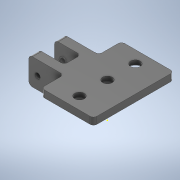
# Autodesk Inventor part: pulleysupport2
Saved by Autodesk Inventor 2020.2 (Build 242310000, 310)
## iProperties
Created: 2020-08-06
Part Number: pulleysupport2
Material: Generic
Document SubType Name: Modeling
Designer: JK
Density: 1 g/cm^3
Appearance: Smooth - Black
Author: JK
Autodesk Inventor part; units mm, degrees
sketch "Sketch1" plane through (0, 0, 0) normal (0, 1, 0) x (-1, 0, 0)
  line L0 (-15, 23) -> (15, 23)
  line L1 (15, 23) -> (15, -23)
  line L2 (15, -23) -> (-15, -23)
  line L3 (-15, -23) -> (-15, 23)
  line L4 (-15, 23) -> (15, -23) construction
  line L5 (15, 23) -> (-15, -23) construction
  circle A0 centre (0, 16) radius 1.75
  circle A1 centre (0, -16) radius 1.75
  point P0 (0, 0)
  dimension "d0" = 3.5
  dimension "d1" = 30
  dimension "d2" = 46
  dimension "d3" = 16
  dimension "d4" = 16
  constraints: 12 end point, 2 centre point, 2 midpoint, 2 parallel, 1 equal radius, 1 horizontal, 1 perpendicular
  measures "d0" diameter of A0
  measures "d1" distance of L0.start L0.end
  measures "d2" distance of L0.end L1.end
  measures "d3" distance of A0.centre point (0, 0)
  measures "d4" distance of A1.centre point (0, 0)
extrude "Extrusion1" add sketch "Sketch1" along normal blind 4
sketch "Sketch2" plane through (0, 4, 0) normal (0, 1, 0) x (1, 0, 0)
  line L0 (15, -23) -> (15, 23) projected
  line L1 (15, -10) -> (-35, -10)
  line L2 (-35, -10) -> (-35, 10)
  line L3 (-35, 10) -> (15, 10)
  line L4 (15, 10) -> (15, -10)
  line L5 (-15, -23) -> (15, -23) projected
  point P0 (0, 0)
  point P1 (15, 10)
  dimension "d9" = 20
  dimension "d11" = 10
  dimension "d28" = 50
  constraints: 8 end point, 2 parallel, 1 horizontal, 1 perpendicular, 1 point on line
  measures "d9" distance between parallel lines of L1 L3
  measures "d11" distance from line of L1 point (0, 0)
  measures "d28" distance between parallel lines of L0 L2
extrude "Extrusion2" add sketch "Sketch2" against normal blind 20
sketch "Sketch3" plane through (0, -16, 0) normal (0, -1, 0) x (1, 0, 0)
  point P0 (0, 0)
sketch "Sketch4" plane through (0, -16, 0) normal (0, -1, 0) x (1, 0, 0)
  line L0 (35.8206, -4.75) -> (-35.8206, -4.75)
  line L1 (-35.8206, -4.75) -> (-35.8206, 4.75)
  line L2 (-35.8206, 4.75) -> (35.8206, 4.75)
  line L3 (35.8206, 4.75) -> (35.8206, -4.75)
  line L4 (35.8206, -4.75) -> (-35.8206, 4.75) construction
  line L5 (-35.8206, -4.75) -> (35.8206, 4.75) construction
  point P0 (0, 0)
  dimension "d12" = 9.5
  constraints: 12 end point, 2 midpoint, 2 parallel, 1 horizontal, 1 perpendicular
  measures "d12" distance between parallel lines of L2 L0
extrude "Extrusion3" cut sketch "Sketch4" against normal up to surface (16 mm away)
sketch "Sketch5" plane through (-15, 4, -10) normal (0, 0, -1) x (-1, 0, 0)
  circle A0 centre (15, -8) radius 1.5
  line L0 (20, 0) -> (20, -20) projected
  line L1 (20, -20) -> (-30, -20) projected
  line L2 (20, 0) -> (0, 0) projected
  point P0 (-15, -4)
  dimension "d15" = 3
  dimension "d16" = 5
  dimension "d49" = 8
  constraints: 1 centre point
  measures "d15" diameter of A0
  measures "d16" distance from line of L0 A0.centre
  measures "d49" distance from line of A0.centre L2
extrude "Extrusion4" cut sketch "Sketch5" against normal through all
sketch "Sketch6" plane through (0, 0, 0) normal (0, -1, 0) x (1, 0, 0)
  circle A0 centre (0, -16) radius 1.75 projected
  circle A1 centre (0, -16) radius 4.75
  circle A2 centre (0, 16) radius 1.75 projected
  circle A3 centre (0, 16) radius 4.75
  point P0 (0, 0)
  dimension "d20" = 9.5
  dimension "d21" = 9.5
  constraints: 2 centre point, 2 coincident
  measures "d20" diameter of A1
  measures "d21" diameter of A3
extrude "Extrusion5" cut sketch "Sketch6" against normal blind 2
fillet "Fillet1" radius 2 6 edges at (-15, 2, -23) (15, 2, -23) (-15, 2, 23) (15, 2, 23) (-35, -16, -7.375) (-35, -16, 7.375)
chamfer "Chamfer1" distance 16 angle 45 2 edges at (15, -16, -7.375) (15, -16, 7.375)
fillet "Fillet2" radius 2 2 edges at (-1, -16, 7.375) (-1, -16, -7.375)
fillet "Fillet4" radius 2 2 edges at (0, 0, 10) (0, 0, -10)
ref_plane "Work Plane2" through (-35, 0, 2.75) normal (0, -1, 0) x (1, 0, 0)
sketch "Sketch8" plane through (-35, 0, 2.75) normal (0, -1, 0) x (1, 0, 0)
  circle A0 centre (35, -2.75) radius 4.75
  dimension "d32" = 9.5
  constraints: 1 centre point, 1 coincident
  measures "d32" diameter of A0
extrude "Extrusion6" cut sketch "Sketch8" along normal blind 20.5 and the other way blind 2
ref_plane "Work Plane3" through (0, 2, 0) normal (0, -1, 0) x (1, 0, 0)
sketch "Sketch9" plane through (0, 2, 0) normal (0, -1, 0) x (1, 0, 0)
  circle A0 centre (0, 0) radius 2.75
  circle A1 centre (0, -16) radius 1.75 projected
  circle A2 centre (0, -16) radius 2.75
  circle A3 centre (0, 16) radius 1.75 projected
  circle A4 centre (0, 16) radius 2.75
  dimension "d37" = 5.5
  constraints: 3 centre point, 3 coincident, 2 equal radius
  measures "d37" diameter of A0
extrude "Extrusion7" cut sketch "Sketch9" against normal blind 10
sketch "Sketch10" plane through (-1.8284, -16, 4.75) normal (0, 0, -1) x (-1, 0, 0)
  circle A0 centre (28.1716, 12) radius 1.5 projected
  circle A1 centre (28.1716, 12) radius 2.15
  point P0 (-1.8284, 16)
  dimension "d40" = 4.3
  constraints: 1 centre point, 1 coincident
  measures "d40" diameter of A1
extrude "Extrusion8" add sketch "Sketch10" along normal blind 10
sketch "Sketch11" plane through (0, -16, 0) normal (0, -1, 0) x (1, 0, 0)
  line L0 (-37.4178, 4.35) -> (-15.1457, 4.35)
  line L1 (-15.1457, 4.35) -> (-15.1457, -4.35)
  line L2 (-15.1457, -4.35) -> (-37.4178, -4.35)
  line L3 (-37.4178, -4.35) -> (-37.4178, 4.35)
  line L4 (-33, 4.75) -> (-1.8284, 4.75) projected
  line L5 (-1.8284, -4.75) -> (-33, -4.75) projected
  point P0 (0, 0)
  dimension "d45" = 0.4
  dimension "d46" = 0.4
  constraints: 8 end point, 2 parallel, 1 horizontal, 1 perpendicular
  measures "d45" distance between parallel lines of L4 L0
  measures "d46" distance between parallel lines of L5 L2
extrude "Extrusion9" cut sketch "Sketch11" against normal blind 14.75
ref_plane "Work Plane1" through (-35, 0, -2.75) normal (0, -1, 0) x (1, 0, 0)
sketch "Sketch12" plane through (-35, 0, -2.75) normal (0, -1, 0) x (1, 0, 0)
  line L0 (35, 7.5) -> (5.789, 7.5) projected
  line L1 (0, -2) -> (2, -2) projected
  line L2 (15, 7.5) -> (0, 7.5)
  line L3 (0, 7.5) -> (0, -2)
  line L4 (0, -2) -> (15, -2)
  line L5 (15, -2) -> (15, 7.5)
  point P0 (35, 2.75)
  dimension "d50" = 15
  constraints: 8 end point, 2 parallel, 1 horizontal, 1 perpendicular, 1 point on line
  measures "d50" distance between parallel lines of L5 L3
extrude "Extrusion10" cut sketch "Sketch12" against normal through all
sketch "Sketch13" plane through (0, -16, 0) normal (0, -1, 0) x (1, 0, 0)
  line L0 (13, -10) -> (-15, -10) projected
  line L1 (-15, 10) -> (-15, 21) projected
  line L2 (-9.2716, -10) -> (-15, -10)
  line L3 (-15, -10) -> (-15, 10)
  line L4 (-15, 10) -> (-9.2716, 10)
  line L5 (-9.2716, 10) -> (-9.2716, -10)
  point P0 (0, 0)
  point P1 (-15, -10)
  constraints: 8 end point, 2 parallel, 1 horizontal, 1 perpendicular, 1 point on line
extrude "Extrusion11" add sketch "Sketch13" against normal up to surface (16 mm away)
fillet "Fillet5" radius 2 4 edges at (-35, 4, -7.375) (-35, 4, 7.375) (-15, 1, -10) (-15, 1, 10)
sketch "Sketch14" plane through (0, -16, 0) normal (0, -1, 0) x (1, 0, 0)
  line L0 (18.783, 13.4678) -> (-42.7613, 13.4678)
  line L1 (-42.7613, 13.4678) -> (-42.7613, -13.4678)
  line L2 (-42.7613, -13.4678) -> (18.783, -13.4678)
  line L3 (18.783, -13.4678) -> (18.783, 13.4678)
  line L4 (18.783, 13.4678) -> (-42.7613, -13.4678) construction
  line L5 (-42.7613, 13.4678) -> (18.783, -13.4678) construction
  point P0 (0, 0)
  point P1 (-11.9891, 0)
  constraints: 12 end point, 2 midpoint, 2 parallel, 1 horizontal, 1 perpendicular
extrude "Extrusion12" cut sketch "Sketch14" against normal blind 5
fillet "Fillet6" radius 2 4 edges at (4, -11, -7.375) (4, -11, 7.375) (-35, -11, -7.375) (-35, -11, 7.375)
sketch "Sketch15" plane through (0, -11, 0) normal (0, -1, 0) x (1, 0, 0)
  line L0 (-20, 4.75) -> (-20, -4.75) projected
  line L1 (-15, -4.75) -> (-15, 4.75) projected
  line L2 (-20, -4.75) -> (-15, -4.75)
  line L3 (-15, -4.75) -> (-15, 4.75)
  line L4 (-15, 4.75) -> (-20, 4.75)
  line L5 (-20, 4.75) -> (-20, -4.75)
  point P0 (0, 0)
  constraints: 8 end point, 2 parallel, 1 horizontal, 1 perpendicular
extrude "Extrusion13" add sketch "Sketch15" against normal up to surface (11 mm away)
fillet "Fillet7" radius 2 4 edges at (-20, -3.5, -4.75) (-20, -3.5, 4.75) (-9.2716, -5.5, -4.75) (-9.2716, -5.5, 4.75)
body "Solid1"
